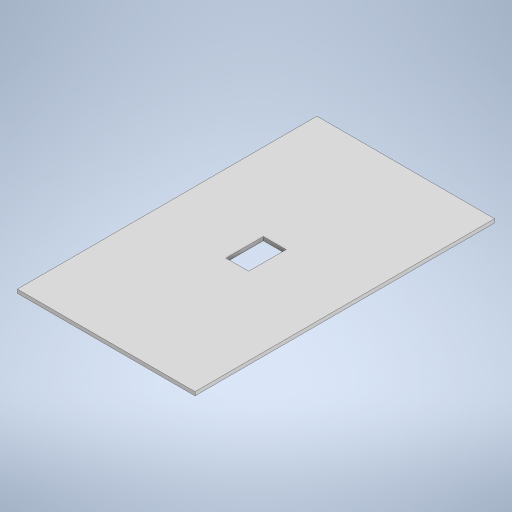
# Autodesk Inventor part: TapaBaterias
Saved by Autodesk Inventor 2024 (Build 280153000, 153)
## iProperties
Created: 2024-07-14
Part Number: TapaBaterias
Material: Genérico
Document SubType Name: Modeling
Designer: sergi
Density: 1 g/cm^3
Appearance: Valor por defecto
Author: sergi
Autodesk Inventor part; units mm, degrees
ref_plane "YZ Plane" through (0, 0, 0) normal (1, 0, 0) x (0, 1, 0)
ref_plane "XZ Plane" through (0, 0, 0) normal (0, 1, 0) x (-1, 0, 0)
ref_plane "XY Plane" through (0, 0, 0) normal (0, 0, 1) x (1, 0, 0)
sketch "Boceto1" plane through (0, 0, 0) normal (0, 1, 0) x (-1, 0, 0)
  line L0 (-24.25, -40.9) -> (24.25, -40.9)
  line L1 (24.25, -40.9) -> (24.25, 40.9)
  line L2 (24.25, 40.9) -> (-24.25, 40.9)
  line L3 (-24.25, 40.9) -> (-24.25, -40.9)
  line L4 (-24.25, -40.9) -> (24.25, 40.9) construction
  line L5 (24.25, -40.9) -> (-24.25, 40.9) construction
  point P0 (0, 0)
  dimension "d0" = 48.5
  dimension "d1" = 81.8
  constraints: 12 end point, 2 midpoint, 2 parallel, 1 horizontal, 1 perpendicular
  measures "d0" distance of L2.end L1.end
  measures "d1" distance of L1.end L0.end
extrude "Extrusión1" add sketch "Boceto1" along normal blind 1
sketch "Boceto2" plane through (0, 1, 0) normal (0, 1, 0) x (1, 0, 0)
  line L0 (3.1, 5.1) -> (-3.1, 5.1)
  line L1 (-3.1, 5.1) -> (-3.1, -5.1)
  line L2 (-3.1, -5.1) -> (3.1, -5.1)
  line L3 (3.1, -5.1) -> (3.1, 5.1)
  line L4 (3.1, 5.1) -> (-3.1, -5.1) construction
  line L5 (-3.1, 5.1) -> (3.1, -5.1) construction
  point P0 (0, 0)
  dimension "d4" = 6.2
  dimension "d5" = 10.2
  constraints: 12 end point, 2 midpoint, 2 parallel, 1 horizontal, 1 perpendicular
  measures "d4" distance of L2.end L1.end
  measures "d5" distance of L1.end L0.end
extrude "Extrusión2" cut sketch "Boceto2" against normal blind 1
